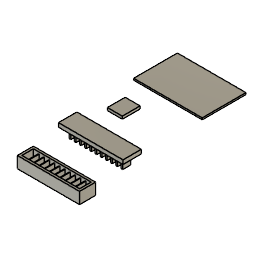
PlanC v1 (Autodesk Fusion 360 design; units mm, degrees)
Autodesk Fusion 360 part; units mm, degrees
note: some values were not read from the file. Chosen so that the rebuilt part matches the saved one: which bodies a step acts on; which face or edge a step refers to.
sketch "Sketch1" plane through (0, 0, 0) normal (0, 0, 1) x (1, 0, 0)
  line L0 (-10, 25) -> (-2, 25)
  line L1 (-2, 25) -> (-2, 5)
  line L2 (-2, 5) -> (-10, 5)
  line L3 (-10, 5) -> (-10, 25)
  line L4 (-7.5, 22) -> (-4.5, 22)
  line L5 (-4.5, 22) -> (-4.5, 8)
  line L6 (-4.5, 8) -> (-7.5, 8)
  line L7 (-7.5, 8) -> (-7.5, 22)
  dimension "d1" = 20
  dimension "d2" = 8
  dimension "d3" = 2.5
  dimension "d4" = 2.5
  dimension "d5" = 3
  dimension "d6" = 3
  constraint horizontal L0
  constraint vertical L1
  constraint horizontal L2
  constraint vertical L3
  constraint horizontal L4
  constraint vertical L5
  constraint horizontal L6
  constraint vertical L7
  measures "d1" distance of L0.start L2.end
  measures "d2" distance of L0.start L0.end
  measures "d3" distance of L1 L5
  measures "d4" distance of L3 L7
  measures "d5" distance of L2 L6
  measures "d6" distance of L0 L4
extrude "Extrude1" add sketch "Sketch1" against normal blind 20 contours L0 L1 L2 L3 | L4 L5 L6 L7 makes body 1
extrude "Extrude2" cut sketch "Sketch1" against normal blind 18 contours L4 L5 L6 L7 bodies 1
sketch "Sketch2" plane through (-2, 0, 0) normal (1, 0, 0) x (0, 1, 0)
  line L0 (25, 0) -> (5, 0)
  line L1 (5, 0) -> (5, -20)
  line L2 (5, -20) -> (25, -20)
  line L3 (25, -20) -> (25, 0)
  line L4 (25, -3) -> (5, -3)
  line L5 (5, -3) -> (5, 0)
  line L6 (5, 0) -> (25, 0)
  line L7 (25, 0) -> (25, -3)
  dimension "d11" = 3
  constraint horizontal L4
  constraint vertical L5
  constraint horizontal L6
  constraint vertical L7
  constraint coincident L0.end L1.start
  constraint coincident L3 L4.start
  measures "d11" distance of L4.start L0.start
extrude "Extrude3" add sketch "Sketch2" along normal blind 1 contours L0 L1 L3 L4 L5 L6 L7 bodies 1
pattern_linear "R-Pattern1" count 11 spacing 9 along (1, 0, 0) of bodies 1 makes body 2 at (-1, 11.6667, -6.6667) makes body 3 at (8, 11.6667, -6.6667) makes body 4 at (17, 11.6667, -6.6667) makes body 5 at (26, 11.6667, -6.6667) makes body 6 at (35, 11.6667, -6.6667) makes body 7 at (44, 11.6667, -6.6667) makes body 8 at (53, 11.6667, -6.6667) makes body 9 at (62, 11.6667, -6.6667) makes body 10 at (71, 11.6667, -6.6667) makes body 11 at (80, 11.6667, -6.6667)
combine "Combine1" operation add target body 6 tool bodies 7 1 2 5 4 11 8 3 10 9
move_face "OffsetFaces1" offset 1 1 faces at (88, 18.3333, -8.6667) on bodies 6
move_face "OffsetFaces2" offset 1 1 faces at (-10, 18.3333, -13.3333) on bodies 6
sketch "Sketch3" plane through (0, 0, 0) normal (0, 0, 1) x (-1, 0, 0)
  line L0 (4.5, -22) -> (4.5, -8)
  line L1 (4.5, -8) -> (7.5, -8)
  line L2 (7.5, -8) -> (7.5, -22)
  line L3 (7.5, -22) -> (4.5, -22)
  line L4 (-4.5, -22) -> (-4.5, -8)
  line L5 (-4.5, -8) -> (-1.5, -8)
  line L6 (-1.5, -8) -> (-1.5, -22)
  line L7 (-1.5, -22) -> (-4.5, -22)
  line L8 (-13.5, -22) -> (-13.5, -8)
  line L9 (-13.5, -8) -> (-10.5, -8)
  line L10 (-10.5, -8) -> (-10.5, -22)
  line L11 (-10.5, -22) -> (-13.5, -22)
  line L12 (-58.5, -22) -> (-58.5, -8)
  line L13 (-58.5, -8) -> (-55.5, -8)
  line L14 (-55.5, -8) -> (-55.5, -22)
  line L15 (-55.5, -22) -> (-58.5, -22)
  line L16 (-22.5, -22) -> (-22.5, -8)
  line L17 (-22.5, -8) -> (-19.5, -8)
  line L18 (-19.5, -8) -> (-19.5, -22)
  line L19 (-19.5, -22) -> (-22.5, -22)
  line L20 (-31.5, -22) -> (-31.5, -8)
  line L21 (-31.5, -8) -> (-28.5, -8)
  line L22 (-28.5, -8) -> (-28.5, -22)
  line L23 (-28.5, -22) -> (-31.5, -22)
  line L24 (-49.5, -22) -> (-49.5, -8)
  line L25 (-49.5, -8) -> (-46.5, -8)
  line L26 (-46.5, -8) -> (-46.5, -22)
  line L27 (-46.5, -22) -> (-49.5, -22)
  line L28 (-40.5, -22) -> (-40.5, -8)
  line L29 (-40.5, -8) -> (-37.5, -8)
  line L30 (-37.5, -8) -> (-37.5, -22)
  line L31 (-37.5, -22) -> (-40.5, -22)
  line L32 (-67.5, -22) -> (-67.5, -8)
  line L33 (-67.5, -8) -> (-64.5, -8)
  line L34 (-64.5, -8) -> (-64.5, -22)
  line L35 (-64.5, -22) -> (-67.5, -22)
  line L36 (-76.5, -22) -> (-76.5, -8)
  line L37 (-76.5, -8) -> (-73.5, -8)
  line L38 (-73.5, -8) -> (-73.5, -22)
  line L39 (-73.5, -22) -> (-76.5, -22)
  line L40 (-85.5, -22) -> (-85.5, -8)
  line L41 (-85.5, -8) -> (-82.5, -8)
  line L42 (-82.5, -8) -> (-82.5, -22)
  line L43 (-82.5, -22) -> (-85.5, -22)
  line L44 (11, -5) -> (-89, -5)
  line L45 (-89, -5) -> (-89, -25)
  line L46 (-89, -25) -> (11, -25)
  line L47 (11, -25) -> (11, -5)
  line L48 (-82.5, -19.5146) -> (4.5, -19.5146)
  line L49 (4.5, -19.5146) -> (4.5, -10.4854)
  line L50 (4.5, -10.4854) -> (-82.5, -10.4854)
  line L51 (-82.5, -10.4854) -> (-82.5, -19.5146)
  line L52 (-82.5, -13.9962) -> (4.5, -13.9962)
  line L53 (-82.5, -15.9962) -> (4.5, -15.9962)
  line L54 (4.5, -15.9962) -> (4.5, -13.9962)
  line L55 (-82.5, -15.9962) -> (-82.5, -13.9962)
  dimension "d20" = 2
  constraint horizontal L48
  constraint vertical L49
  constraint horizontal L50
  constraint vertical L51
  constraint coincident L0 L49.end
  constraint coincident L42 L48.start
  constraint midpoint L42 L51
  constraint coincident L51 L52.start
  constraint coincident L42 L53.start
  constraint coincident L49 L52.end
  constraint parallel L50 L52
  constraint coincident L49 L53.end
  constraint parallel L48 L53
  measures "d20" distance of L52 L53
extrude "Extrude4" cut sketch "Sketch3" against normal blind 2 contours L0 L6 L49 L52 L53 L54 | L4 L6 L52 L53 | L4 L10 L52 L53 | L8 L10 L52 L53 | L8 L18 L52 L53 | L16 L18 L52 L53 | L16 L22 L52 L53 | L20 L22 L52 L53 | L20 L30 L52 L53 | L28 L30 L52 L53 | L26 L28 L52 L53 | L24 L26 L52 L53 | L14 L24 L52 L53 | L12 L14 L52 L53 | L12 L34 L52 L53 | L32 L34 L52 L53 | L32 L38 L52 L53 | L36 L38 L52 L53 | L36 L42 L51 L52 L53 L55 bodies 6
sketch "Sketch4" plane through (0, 0, 0) normal (0, 0, 1) x (-1, 0, 0)
  line L0 (-64.5, -13.9962) -> (-58.5, -13.9962)
  line L1 (-58.5, -13.9962) -> (-58.5, -8)
  line L2 (-58.5, -8) -> (-55.5, -8)
  line L3 (-55.5, -8) -> (-55.5, -13.9962)
  line L4 (-55.5, -13.9962) -> (-49.5, -13.9962)
  line L5 (-49.5, -13.9962) -> (-49.5, -8)
  line L6 (-49.5, -8) -> (-46.5, -8)
  line L7 (-46.5, -8) -> (-46.5, -13.9962)
  line L8 (-46.5, -13.9962) -> (-40.5, -13.9962)
  line L9 (-40.5, -13.9962) -> (-40.5, -8)
  line L10 (-40.5, -8) -> (-37.5, -8)
  line L11 (-37.5, -8) -> (-37.5, -13.9962)
  line L12 (-37.5, -13.9962) -> (-31.5, -13.9962)
  line L13 (-31.5, -13.9962) -> (-31.5, -8)
  line L14 (-31.5, -8) -> (-28.5, -8)
  line L15 (-28.5, -8) -> (-28.5, -13.9962)
  line L16 (-28.5, -13.9962) -> (-22.5, -13.9962)
  line L17 (-22.5, -13.9962) -> (-22.5, -8)
  line L18 (-22.5, -8) -> (-19.5, -8)
  line L19 (-19.5, -8) -> (-19.5, -13.9962)
  line L20 (-19.5, -13.9962) -> (-13.5, -13.9962)
  line L21 (-13.5, -13.9962) -> (-13.5, -8)
  line L22 (-13.5, -8) -> (-10.5, -8)
  line L23 (-10.5, -8) -> (-10.5, -13.9962)
  line L24 (-10.5, -13.9962) -> (-4.5, -13.9962)
  line L25 (-4.5, -13.9962) -> (-4.5, -8)
  line L26 (-4.5, -8) -> (-1.5, -8)
  line L27 (-1.5, -8) -> (-1.5, -13.9962)
  line L28 (-1.5, -13.9962) -> (4.5, -13.9962)
  line L29 (4.5, -13.9962) -> (4.5, -8)
  line L30 (4.5, -8) -> (7.5, -8)
  line L31 (7.5, -8) -> (7.5, -22)
  line L32 (7.5, -22) -> (4.5, -22)
  line L33 (4.5, -22) -> (4.5, -15.9962)
  line L34 (4.5, -15.9962) -> (-1.5, -15.9962)
  line L35 (-1.5, -15.9962) -> (-1.5, -22)
  line L36 (-1.5, -22) -> (-4.5, -22)
  line L37 (-4.5, -22) -> (-4.5, -15.9962)
  line L38 (-4.5, -15.9962) -> (-10.5, -15.9962)
  line L39 (-10.5, -15.9962) -> (-10.5, -22)
  line L40 (-10.5, -22) -> (-13.5, -22)
  line L41 (-13.5, -22) -> (-13.5, -15.9962)
  line L42 (-13.5, -15.9962) -> (-19.5, -15.9962)
  line L43 (-19.5, -15.9962) -> (-19.5, -22)
  line L44 (-19.5, -22) -> (-22.5, -22)
  line L45 (-22.5, -22) -> (-22.5, -15.9962)
  line L46 (-22.5, -15.9962) -> (-28.5, -15.9962)
  line L47 (-28.5, -15.9962) -> (-28.5, -22)
  line L48 (-28.5, -22) -> (-31.5, -22)
  line L49 (-31.5, -22) -> (-31.5, -15.9962)
  line L50 (-31.5, -15.9962) -> (-37.5, -15.9962)
  line L51 (-37.5, -15.9962) -> (-37.5, -22)
  line L52 (-37.5, -22) -> (-40.5, -22)
  line L53 (-40.5, -22) -> (-40.5, -15.9962)
  line L54 (-40.5, -15.9962) -> (-46.5, -15.9962)
  line L55 (-46.5, -15.9962) -> (-46.5, -22)
  line L56 (-46.5, -22) -> (-49.5, -22)
  line L57 (-49.5, -22) -> (-49.5, -15.9962)
  line L58 (-49.5, -15.9962) -> (-55.5, -15.9962)
  line L59 (-55.5, -15.9962) -> (-55.5, -22)
  line L60 (-55.5, -22) -> (-58.5, -22)
  line L61 (-58.5, -22) -> (-58.5, -15.9962)
  line L62 (-58.5, -15.9962) -> (-64.5, -15.9962)
  line L63 (-64.5, -15.9962) -> (-64.5, -22)
  line L64 (-64.5, -22) -> (-67.5, -22)
  line L65 (-67.5, -22) -> (-67.5, -15.9962)
  line L66 (-67.5, -15.9962) -> (-73.5, -15.9962)
  line L67 (-73.5, -15.9962) -> (-73.5, -22)
  line L68 (-73.5, -22) -> (-76.5, -22)
  line L69 (-76.5, -22) -> (-76.5, -15.9962)
  line L70 (-76.5, -15.9962) -> (-82.5, -15.9962)
  line L71 (-82.5, -15.9962) -> (-82.5, -22)
  line L72 (-82.5, -22) -> (-85.5, -22)
  line L73 (-85.5, -22) -> (-85.5, -8)
  line L74 (-85.5, -8) -> (-82.5, -8)
  line L75 (-82.5, -8) -> (-82.5, -13.9962)
  line L76 (-82.5, -13.9962) -> (-76.5, -13.9962)
  line L77 (-76.5, -13.9962) -> (-76.5, -8)
  line L78 (-76.5, -8) -> (-73.5, -8)
  line L79 (-73.5, -8) -> (-73.5, -13.9962)
  line L80 (-73.5, -13.9962) -> (-67.5, -13.9962)
  line L81 (-67.5, -13.9962) -> (-67.5, -8)
  line L82 (-67.5, -8) -> (-64.5, -8)
  line L83 (-64.5, -8) -> (-64.5, -13.9962)
  line L84 (11, -5) -> (-89, -5)
  line L85 (-89, -5) -> (-89, -25)
  line L86 (-89, -25) -> (11, -25)
  line L87 (11, -25) -> (11, -5)
  line L88 (7.5, -22) -> (-85.5, -22)
  line L89 (-85.5, -22) -> (-85.5, -8)
  line L90 (-85.5, -8) -> (7.5, -8)
  line L91 (7.5, -8) -> (7.5, -22)
  line L92 (-86.5, -7) -> (8.5, -7)
  line L93 (8.5, -7) -> (8.5, -23)
  line L94 (8.5, -23) -> (-86.5, -23)
  line L95 (-86.5, -23) -> (-86.5, -7)
  dimension "d23" = -1
  constraint horizontal L88
  constraint vertical L89
  constraint horizontal L90
  constraint vertical L91
  constraint coincident L73.end L74.start
  constraint coincident L31.end L32.start
extrude "Extrude5" add sketch "Sketch4" along normal blind 2 contours L92 L93 L94 L95 bodies 6
sketch "Sketch5" plane through (0, 0, 0) normal (0, 0, 1) x (-1, 0, 0)
  line L0 (-86.5, -23) -> (-86.5, -7)
  line L1 (-86.5, -7) -> (8.5, -7)
  line L2 (8.5, -7) -> (8.5, -23)
  line L3 (8.5, -23) -> (-86.5, -23)
  line L4 (11, -5) -> (-89, -5)
  line L5 (-89, -5) -> (-89, -25)
  line L6 (-89, -25) -> (11, -25)
  line L7 (11, -25) -> (11, -5)
  line L8 (-82.5, -22) -> (-76.5, -22)
  line L9 (-76.5, -22) -> (-76.5, -16)
  line L10 (-76.5, -16) -> (-82.5, -16)
  line L11 (-82.5, -16) -> (-82.5, -22)
  line L12 (-76.5, -14) -> (-82.5, -14)
  line L13 (-82.5, -14) -> (-82.5, -8)
  line L14 (-82.5, -8) -> (-76.5, -8)
  line L15 (-76.5, -8) -> (-76.5, -14)
  line L16 (-81.5, -13) -> (-81.5, -9)
  line L17 (-81.5, -9) -> (-77.5, -9)
  line L18 (-77.5, -9) -> (-77.5, -13)
  line L19 (-77.5, -13) -> (-81.5, -13)
  line L20 (-81.5, -17) -> (-81.5, -21)
  line L21 (-81.5, -21) -> (-77.5, -21)
  line L22 (-77.5, -21) -> (-77.5, -17)
  line L23 (-77.5, -17) -> (-81.5, -17)
  dimension "d26" = 1
  dimension "d27" = -1
  constraint horizontal L8
  constraint vertical L9
  constraint horizontal L10
  constraint vertical L11
  constraint horizontal L12
  constraint vertical L13
  constraint horizontal L14
  constraint vertical L15
extrude "Extrude6" add sketch "Sketch5" along normal blind 2 separate body contours L16 L17 L18 L19 | L20 L21 L22 L23 makes body 12 at (80.1667, 18.3333, 0) makes body 13 at (80.1667, 10.3333, 0)
pattern_linear "R-Pattern2" count 10 spacing 9 along (-1, 0, 0) of bodies 12 13 makes body 14 at (71.1667, 18.3333, 0) makes body 15 at (62.1667, 18.3333, 0) makes body 16 at (53.1667, 18.3333, 0) makes body 17 at (44.1667, 18.3333, 0) makes body 18 at (35.1667, 18.3333, 0) makes body 19 at (26.1667, 18.3333, 0) makes body 20 at (17.1667, 18.3333, 0) makes body 21 at (8.1667, 18.3333, 0) makes body 22 at (-0.8333, 18.3333, 0) makes body 23 at (71.1667, 10.3333, 0) makes body 24 at (62.1667, 10.3333, 0) makes body 25 at (53.1667, 10.3333, 0) makes body 26 at (44.1667, 10.3333, 0) makes body 27 at (35.1667, 10.3333, 0) makes body 28 at (26.1667, 10.3333, 0) makes body 29 at (17.1667, 10.3333, 0) makes body 30 at (8.1667, 10.3333, 0) makes body 31 at (-0.8333, 10.3333, 0)
combine "Combine2" operation add target body 6 tool bodies 16 27 18 23 13 25 24 30 31 14 20 21 22 26 28 19 12 29 17 15
copy_body "CopyPasteBodies1" bodies 6 makes body 32
move_body "Move1" bodies 32 to x (1, 0, 0) y (0, 1, 0) z (0, 0, 1) at (0, 0, 0)
move_body "Move2" bodies 32 to x (1, 0, 0) y (0, 1, 0) z (0, 0, 1) at (-0.0659, 29.5076, 0.0387)
ref_plane "WorkPlane1" through (52.5, 19, 22) normal (0, 0, 1) x (1, 0, 0)
sketch "Sketch6" plane through (0, 0, 22) normal (0, 0, 1) x (1, 0, 0)
  line L0 (-18.3939, 63.8464) -> (94.6061, 63.8464)
  line L1 (94.6061, 63.8464) -> (94.6061, -6.1536)
  line L2 (94.6061, -6.1536) -> (-18.3939, -6.1536)
  line L3 (-18.3939, -6.1536) -> (-18.3939, 63.8464)
  dimension "d35" = 113
  dimension "d36" = 70
  constraint horizontal L0
  constraint vertical L1
  constraint horizontal L2
  constraint vertical L3
  measures "d35" distance of L0.start L0.end
  measures "d36" distance of L0.end L1.end
extrude "Extrude7" add sketch "Sketch6" along normal blind 1 separate body makes body 33
copy_body "CopyPasteBodies2" bodies 33 makes body 34
move_body "Move3" bodies 34 to x (1, 0, 0) y (0, 1, 0) z (0, 0, 1) at (-2.0102, 0.9041, 8.7778)
sketch "Sketch7" plane through (0, 0, 0) normal (0, 0, 1) x (1, 0, 0)
  line L0 (0, -25) -> (-20, -25)
  line L1 (-20, -25) -> (-20, -50)
  line L2 (-20, -50) -> (0, -50)
  line L3 (0, -50) -> (0, -25)
  dimension "d41" = 20
  dimension "d42" = 25
  constraint horizontal L0
  constraint vertical L1
  constraint horizontal L2
  constraint vertical L3
  measures "d41" distance of L0.start L0.end
  measures "d42" distance of L0.start L2.end
move_body "Move4" bodies 6 to x (1, 0, 0) y (0, 1, 0) z (0, 0, 1) at (-0.9683, -7.9398, 0)
move_body "Move5" bodies 32 to x (1, 0, 0) y (0, 1, 0) z (0, 0, 1) at (-1.5492, 4.8413, 0)
extrude "Extrude8" add sketch "Sketch7" against normal blind 2.5 separate body makes body 35
sketch "Sketch8" plane through (0, 0, 0) normal (0, 0, 1) x (-1, 0, 0)
  line L0 (0, 50) -> (0, 25)
  line L1 (0, 25) -> (20, 25)
  line L2 (20, 25) -> (20, 50)
  line L3 (20, 50) -> (0, 50)
  circle A0 centre (2, 48) radius 0.75
  circle A1 centre (4, 48) radius 0.75
  circle A2 centre (6, 48) radius 0.75
  circle A3 centre (8, 48) radius 0.75
  circle A4 centre (10, 48) radius 0.75
  circle A5 centre (12, 48) radius 0.75
  circle A6 centre (14, 48) radius 0.75
  circle A7 centre (16, 48) radius 0.75
  circle A8 centre (18, 48) radius 0.75
  circle A9 centre (2, 46) radius 0.75
  circle A10 centre (4, 46) radius 0.75
  circle A11 centre (6, 46) radius 0.75
  circle A12 centre (8, 46) radius 0.75
  circle A13 centre (10, 46) radius 0.75
  circle A14 centre (12, 46) radius 0.75
  circle A15 centre (14, 46) radius 0.75
  circle A16 centre (16, 46) radius 0.75
  circle A17 centre (18, 46) radius 0.75
  circle A18 centre (2, 44) radius 0.75
  circle A19 centre (4, 44) radius 0.75
  circle A20 centre (6, 44) radius 0.75
  circle A21 centre (8, 44) radius 0.75
  circle A22 centre (10, 44) radius 0.75
  circle A23 centre (12, 44) radius 0.75
  circle A24 centre (14, 44) radius 0.75
  circle A25 centre (16, 44) radius 0.75
  circle A26 centre (18, 44) radius 0.75
  circle A27 centre (2, 42) radius 0.75
  circle A28 centre (4, 42) radius 0.75
  circle A29 centre (6, 42) radius 0.75
  circle A30 centre (8, 42) radius 0.75
  circle A31 centre (10, 42) radius 0.75
  circle A32 centre (12, 42) radius 0.75
  circle A33 centre (14, 42) radius 0.75
  circle A34 centre (16, 42) radius 0.75
  circle A35 centre (18, 42) radius 0.75
  dimension "d45" = 1.5
  dimension "d48" = 2
  dimension "d49" = -2
  measures "d45" diameter of A0
extrude "Extrude9" add sketch "Sketch8" along normal blind 0.25 contours A0 | A1 | A2 | A3 | A4 | A5 | A6 | A7 | A8 | A9 | A10 | A11 | A12 | A13 | A14 | A15 | A16 | A17 | A18 | A19 | A20 | A21 | A22 | A23 | A24 | A25 | A26 | A27 | A28 | A29 | A30 | A31 | A32 | A33 | A34 | A35 bodies 35
sketch "Sketch9" plane through (0, 0, -2.5) normal (0, 0, -1) x (1, 0, 0)
  line L0 (0, 25) -> (0, 50)
  line L1 (0, 50) -> (-20, 50)
  line L2 (-20, 50) -> (-20, 25)
  line L3 (-20, 25) -> (0, 25)
  line L4 (-20, 50) -> (0, 50)
  line L5 (0, 50) -> (0, 25)
  line L6 (0, 25) -> (-20, 25)
  line L7 (-20, 25) -> (-20, 50)
  line L8 (3, 22) -> (-23, 22)
  line L9 (-23, 22) -> (-23, 53)
  line L10 (-23, 53) -> (3, 53)
  line L11 (3, 53) -> (3, 22)
  dimension "d52" = -3
  constraint horizontal L4
  constraint vertical L5
  constraint horizontal L6
  constraint vertical L7
  constraint coincident L0.start L3.end
  constraint coincident L1.end L2.start
extrude "Extrude10" add sketch "Sketch9" against normal up to surface (4.75 mm away) separate body contours L0 L1 L2 L3 L4 L5 L6 L7 | L8 L9 L10 L11 makes body 36
combine "Combine1'" operation cut target body 36 tool bodies 35 keep tools result as body 37 in component "Component"
move_body "Move6" bodies 35 to x (1, 0, 0) y (0, 1, 0) z (0, 0, 1) at (3.4845, 4.9798, -19.257)
move_body "Move7" bodies 36 to x (1, 0, 0) y (0, 1, 0) z (0, 0, 1) at (3.2213, -0.8339, -6.1048)
delete_body "RemoveBody1" bodies 36
sketch "Sketch10" plane through (0, 0, 22) normal (0, 0, -1) x (1, 0, 0)
  line L0 (94.6061, 6.1536) -> (-18.3939, 6.1536)
  line L1 (-18.3939, 6.1536) -> (-18.3939, -63.8464)
  line L2 (-18.3939, -63.8464) -> (94.6061, -63.8464)
  line L3 (94.6061, -63.8464) -> (94.6061, 6.1536)
  line L4 (-18.3939, 6.1536) -> (94.6061, 6.1536)
  line L5 (94.6061, 6.1536) -> (94.6061, -63.8464)
  line L6 (94.6061, -63.8464) -> (-18.3939, -63.8464)
  line L7 (-18.3939, -63.8464) -> (-18.3939, 6.1536)
  line L8 (97.6061, 9.1536) -> (97.6061, -66.8464)
  line L9 (97.6061, -66.8464) -> (-21.3939, -66.8464)
  line L10 (-21.3939, -66.8464) -> (-21.3939, 9.1536)
  line L11 (-21.3939, 9.1536) -> (97.6061, 9.1536)
  dimension "d55" = -3
  constraint horizontal L4
  constraint vertical L5
  constraint horizontal L6
  constraint vertical L7
  constraint coincident L2.end L3.start
  constraint coincident L0.end L1.start
extrude "Extrude11" add sketch "Sketch10" against normal up to surface (3 mm away) separate body contours L0 L1 L2 L3 L4 L5 L6 L7 | L8 L9 L10 L11 makes body 38
combine "Combine1''" operation cut target body 38 tool bodies 33 keep tools result as body 39 in component "Component'"
move_body "Move8" bodies 33 to x (1, 0, 0) y (0, 1, 0) z (0, 0, 1) at (-15.8222, 21.1262, -66.9067)
move_body "Move9" bodies 38 to x (1, 0, 0) y (0, 1, 0) z (0, 0, 1) at (-23.6161, 14.4831, 24.6964)
delete_body "RemoveBody2" bodies 38
move_body "Move10" bodies 6 to x (1, 0, 0) y (0, 1, 0) z (0, 0, 1) at (4.4958, -138.4271, 25.5674)
sketch "Sketch11" plane through (0, 0, 5.5674) normal (0, 0, -1) x (1, 0, 0)
  line L0 (46.5275, 141.3668) -> (38.5275, 141.3668)
  line L1 (38.5275, 141.3668) -> (38.5275, 121.3668)
  line L2 (38.5275, 121.3668) -> (46.5275, 121.3668)
  line L3 (46.5275, 121.3668) -> (46.5275, 141.3668)
  line L4 (-7.4179, 121.3668) -> (92.5156, 121.3668)
  line L5 (92.5156, 121.3668) -> (92.5156, 141.3668)
  line L6 (92.5156, 141.3668) -> (-7.4179, 141.3668)
  line L7 (-7.4179, 141.3668) -> (-7.4179, 121.3668)
  line L8 (96.5156, 145.3668) -> (-11.4179, 145.3668)
  line L9 (-11.4179, 145.3668) -> (-11.4179, 117.3668)
  line L10 (-11.4179, 117.3668) -> (96.5156, 117.3668)
  line L11 (96.5156, 117.3668) -> (96.5156, 145.3668)
  dimension "d58" = 4
  constraint horizontal L4
  constraint vertical L5
  constraint horizontal L6
  constraint vertical L7
extrude "Extrude12" add sketch "Sketch11" against normal up to surface (26 mm away) separate body contours L0 L1 L2 L3 L4 L6 | L3 L4 L5 L6 | L1 L4 L6 L7 | L8 L9 L10 L11 makes body 40
combine "Combine3" operation cut target body 40 tool bodies 6 keep tools
move_body "Move11" bodies 6 to x (1, 0, 0) y (0, 1, 0) z (0, 0, 1) at (29.3668, 59.0066, -42.3719)
split "Split1" by plane through (46.5275, -121.3668, 25.5674) normal (0, 0, -1) bodies 40 makes body 41 at (89.0275, -129.0335, 13.5674) makes body 42 at (60.5377, -145.3668, 12.234)
move_body "Move12" bodies 42 to x (1, 0, 0) y (0, 1, 0) z (0, 0, 1) at (-3.0336, -40.3868, 1.7249)
combine "Combine4" operation add target body 41 tool bodies 40
sketch "Sketch12" plane through (0, 0, 31.5674) normal (0, 0, 1) x (-1, 0, 0)
  line L0 (11.4179, 145.3668) -> (-96.5156, 145.3668)
  line L1 (-96.5156, 145.3668) -> (-96.5156, 117.3668)
  line L2 (-96.5156, 117.3668) -> (11.4179, 117.3668)
  line L3 (11.4179, 117.3668) -> (11.4179, 145.3668)
  line L4 (-96.5156, 145.3668) -> (11.4179, 145.3668)
  line L5 (11.4179, 145.3668) -> (11.4179, 117.3668)
  line L6 (11.4179, 117.3668) -> (-96.5156, 117.3668)
  line L7 (-96.5156, 117.3668) -> (-96.5156, 145.3668)
  line L8 (13.4179, 115.3668) -> (-98.5156, 115.3668)
  line L9 (-98.5156, 115.3668) -> (-98.5156, 147.3668)
  line L10 (-98.5156, 147.3668) -> (13.4179, 147.3668)
  line L11 (13.4179, 147.3668) -> (13.4179, 115.3668)
  dimension "d61" = -2
  constraint horizontal L4
  constraint vertical L5
  constraint horizontal L6
  constraint vertical L7
  constraint coincident L2.end L3.start
  constraint coincident L0.end L1.start
extrude "Extrude13" add sketch "Sketch12" against normal up to surface (7 mm away) bodies 41
move_body "Move13" bodies 42 to x (1, 0, 0) y (0, 1, 0) z (0, 0, 1) at (5.4754, -37.3314, -4.9351)
component "Component" placed x (1, 0, 0) y (0, 1, 0) z (0, 0, 1) at (0, 0, 0)
component "Component'" placed x (1, 0, 0) y (0, 1, 0) z (0, 0, 1) at (0, 0, 0)
hidden bodies 6 32 33 34 35
